Curved Piece (Autodesk Fusion 360 design; units mm, degrees)
Autodesk Fusion 360 part; units mm, degrees
sketch "Sketch1" plane through (0, 0, 0) normal (0, 0, 1) x (1, 0, 0)
  spline S0 degree 5 poles (-4.0225, 4.9457) (-4.3832, 4.8836) (-5.0983, 4.7502) (-6.1514, 4.5234) (-7.5163, 4.167) (-9.156, 3.6306) (-10.7265, 3.001) (-12.2235, 2.275) (-13.6402, 1.4484) (-14.9669, 0.5153) (-16.1924, -0.5297) (-17.3048, -1.6899) (-18.293, -2.9647) (-19.1478, -4.3479) (-19.8637, -5.8249) (-20.4387, -7.3761) (-20.8745, -8.9799) (-21.1767, -10.6153) (-21.3553, -12.265) (-21.4247, -13.9182) (-21.402, -15.5694) (-21.3053, -17.2166) (-21.1515, -18.8602) (-20.9547, -20.5013) (-20.7245, -22.1409) (-20.4667, -23.7795) (-20.2409, -25.0897) (-20.0609, -26.072) (-19.9363, -26.7268) (-19.8729, -27.0541) knots 0 0 0 0 0 0 0.04 0.08 0.12 0.16 0.2 0.24 0.28 0.32 0.36 0.4 0.44 0.48 0.52 0.56 0.6 0.64 0.68 0.72 0.76 0.8 0.84 0.88 0.92 0.96 1 1 1 1 1 1
  spline S1 degree 3 poles (-4.3622, 6.9167) (-8.1004, 6.2724) (-11.5169, 5.1) (-14.4993, 3.2309) (-16.7769, 1.8036) (-18.7852, -0.0839) (-20.2589, -2.3858) (-21.8745, -4.9093) (-22.8164, -7.871) (-23.1893, -10.8003) (-23.5774, -13.8492) (-23.3919, -16.8307) (-23.0586, -19.71) (-22.7573, -22.3125) (-22.3334, -24.8713) (-21.8363, -27.4348) knots 0 0 0 0 0.234757 0.234757 0.234757 0.414034 0.414034 0.414034 0.610562 0.610562 0.610562 0.815115 0.815115 0.815115 1 1 1 1
  line L0 (-21.8363, -27.4348) -> (-19.8729, -27.0541)
  line L1 (-4.3622, 6.9167) -> (-4.0225, 4.9457)
  line L2 (-19.8729, -27.0541) -> (-4.0225, 4.9457)
  point P0 (-12.471, 2.1046)
  point P1 (-18.3028, -3.0542)
  point P2 (-21.1439, -10.6056)
  point P3 (-21.1439, -18.8298)
  dimension "d1" = 2
extrude "Extrude1" add sketch "Sketch1" along normal blind 188
extrude "Extrude2" cut sketch "Sketch1" along normal blind 2.2 contours S0 L2
extrude "Extrude3" cut sketch "Sketch1" along normal blind 2 from surface at 186 contours S0 L2
move_face "OffsetFaces1" offset -0.2 1 faces at (-15.4455, -10.109, 186)
